Autodesk Fusion 360 part; units mm, degrees
(part 2 of 3)
  line L695 (-16.549, 126.6806) -> (-16.4532, 126.8438)
  line L696 (-16.4532, 126.8438) -> (-16.3127, 126.9927)
  line L697 (-16.3127, 126.9927) -> (-16.1723, 127.1416)
  line L698 (-16.1723, 127.1416) -> (-16.0457, 127.2313)
  spline S85 degree 3 poles (-16.0457, 127.2313) (-15.8814, 127.3478) (-15.7503, 127.4125) (-15.5307, 127.4855) knots 0 0 0 0 1 1 1 1
  line L699 (-15.5307, 127.4855) -> (-15.3521, 127.5448)
  line L700 (-15.3521, 127.5448) -> (-14.9951, 127.5456)
  line L701 (-14.9951, 127.5456) -> (-14.6381, 127.5465)
  line L702 (-14.6381, 127.5465) -> (-14.4281, 127.4721)
  line L703 (-14.4281, 127.4721) -> (-14.2181, 127.3978)
  line L704 (-14.2181, 127.3978) -> (-8.7577, 124.2519)
  spline S86 degree 3 poles (-8.7577, 124.2519) (-5.7545, 122.5216) (-3.2454, 121.0723) (-3.1819, 121.0312) knots 0 0 0 0 1 1 1 1
  line L705 (-3.1819, 121.0312) -> (-3.0664, 120.9565)
  line L706 (-3.0664, 120.9565) -> (-2.9089, 120.7961)
  line L707 (-2.9089, 120.7961) -> (-2.7514, 120.6356)
  line L708 (-2.7514, 120.6356) -> (-2.6525, 120.4684)
  line L709 (-2.6525, 120.4684) -> (-2.5536, 120.3011)
  line L710 (-2.5536, 120.3011) -> (-2.4864, 120.1016)
  line L711 (-2.4864, 120.1016) -> (-2.4191, 119.9021)
  line L712 (-2.4191, 119.9021) -> (-2.4097, 119.608)
  line L713 (-2.4097, 119.608) -> (-2.4003, 119.314)
  line L714 (-2.4003, 119.314) -> (-2.4444, 119.1292)
  line L715 (-2.4444, 119.1292) -> (-2.4886, 118.9443)
  line L716 (-2.4886, 118.9443) -> (-2.5601, 118.7895)
  spline S87 degree 3 poles (-2.5601, 118.7895) (-2.6533, 118.5878) (-2.7387, 118.4645) (-2.9076, 118.2878) knots 0 0 0 0 1 1 1 1
  line L717 (-2.9076, 118.2878) -> (-3.0454, 118.1436)
  line L718 (-3.0454, 118.1436) -> (-3.1674, 118.0604)
  spline S88 degree 3 poles (-3.1674, 118.0604) (-3.3211, 117.9556) (-3.554, 117.8452) (-3.7174, 117.7997) knots 0 0 0 0 1 1 1 1
  line L719 (-3.7174, 117.7997) -> (-3.8434, 117.7647)
  line L720 (-3.8434, 117.7647) -> (-4.1584, 117.7571)
  line L721 (-4.1584, 117.7571) -> (-4.4735, 117.7496)
  line L722 (-4.4735, 117.7496) -> (-4.625, 117.7904)
  spline S89 degree 3 poles (-3.8806, 117.8246) (-3.6716, 117.8678) (-3.4777, 117.9415) (-3.3069, 118.0427) knots 0 0 0 0 1 1 1 1
  line L723 (-3.3069, 118.0427) -> (-3.1695, 118.1242)
  line L724 (-3.1695, 118.1242) -> (-3.0182, 118.2642)
  line L725 (-3.0182, 118.2642) -> (-2.867, 118.4043)
  line L726 (-2.867, 118.4043) -> (-2.7535, 118.5756)
  line L727 (-2.7535, 118.5756) -> (-2.64, 118.747)
  line L728 (-2.64, 118.747) -> (-2.5873, 118.8731)
  spline S90 degree 3 poles (-2.5873, 118.8731) (-2.5584, 118.9424) (-2.5191, 119.0592) (-2.5001, 119.1327) knots 0 0 0 0 1 1 1 1
  line L729 (-2.5001, 119.1327) -> (-2.4655, 119.2663)
  line L730 (-2.4655, 119.2663) -> (-2.4531, 119.4414)
  line L731 (-2.4531, 119.4414) -> (-2.4407, 119.6165)
  line L732 (-2.4407, 119.6165) -> (-2.4666, 119.7766)
  line L733 (-2.4666, 119.7766) -> (-2.4924, 119.9366)
  line L734 (-2.4924, 119.9366) -> (-2.543, 120.0853)
  spline S91 degree 3 poles (-2.543, 120.0853) (-2.666, 120.4472) (-2.9021, 120.7612) (-3.2134, 120.9768) knots 0 0 0 0 1 1 1 1
  spline S92 degree 3 poles (-3.2134, 120.9768) (-3.2973, 121.035) (-14.1137, 127.2678) (-14.2431, 127.3327) knots 0 0 0 0 1 1 1 1
  spline S93 degree 3 poles (-14.2431, 127.3327) (-14.3718, 127.3971) (-14.5821, 127.4647) (-14.7417, 127.493) knots 0 0 0 0 1 1 1 1
  line L735 (-14.7417, 127.493) -> (-14.8663, 127.515)
  line L736 (-14.8663, 127.515) -> (-15.0042, 127.5148)
  line L737 (-15.0042, 127.5148) -> (-15.1421, 127.5145)
  line L738 (-15.1421, 127.5145) -> (-15.3388, 127.4739)
  line L739 (-15.3388, 127.4739) -> (-15.5355, 127.4333)
  line L740 (-15.5355, 127.4333) -> (-15.7483, 127.3288)
  line L741 (-15.7483, 127.3288) -> (-15.9612, 127.2242)
  line L742 (-15.9612, 127.2242) -> (-16.0864, 127.1225)
  line L743 (-16.0864, 127.1225) -> (-16.2117, 127.0208)
  line L744 (-16.2117, 127.0208) -> (-16.3352, 126.8742)
  line L745 (-16.3352, 126.8742) -> (-16.4587, 126.7275)
  line L746 (-16.4587, 126.7275) -> (-16.5605, 126.5175)
  line L747 (-16.5605, 126.5175) -> (-16.6624, 126.3075)
  line L748 (-16.6624, 126.3075) -> (-16.699, 126.171)
  line L749 (-16.699, 126.171) -> (-16.7357, 126.0344)
  line L750 (-16.7357, 126.0344) -> (-16.7365, 125.7719)
  line L751 (-16.7365, 125.7719) -> (-16.7373, 125.5094)
  line L752 (-16.7373, 125.5094) -> (-16.6987, 125.3624)
  line L753 (-16.6987, 125.3624) -> (-16.6601, 125.2154)
  line L754 (-16.6601, 125.2154) -> (-16.5778, 125.038)
  line L755 (-16.5778, 125.038) -> (-16.4955, 124.8605)
  line L756 (-16.4955, 124.8605) -> (-16.3808, 124.7081)
  line L757 (-16.3808, 124.7081) -> (-16.2661, 124.5557)
  line L758 (-16.2661, 124.5557) -> (-16.1449, 124.455)
  spline S94 degree 3 poles (-16.1449, 124.455) (-16.0783, 124.3997) (-15.9766, 124.3246) (-15.9189, 124.2882) knots 0 0 0 0 1 1 1 1
  spline S95 degree 3 poles (-15.9189, 124.2882) (-15.8613, 124.2519) (-13.3806, 122.8204) (-10.4063, 121.1072) knots 0 0 0 0 1 1 1 1
  line L759 (-10.4063, 121.1072) -> (-4.9985, 117.9923)
  line L760 (-4.9985, 117.9923) -> (-4.841, 117.9247)
  line L761 (-4.841, 117.9247) -> (-4.6835, 117.857)
  line L762 (-4.6835, 117.857) -> (-4.5365, 117.8259)
  line L763 (-4.5365, 117.8259) -> (-4.3895, 117.7949)
  line L764 (-4.3895, 117.7949) -> (-4.2153, 117.7931)
  line L765 (-4.2153, 117.7931) -> (-4.0412, 117.7914)
  line L766 (-4.0412, 117.7914) -> (-3.8806, 117.8246)
  spline S96 degree 3 poles (3.4229, 117.7903) (3.342, 117.8116) (3.2176, 117.8526) (3.1465, 117.8815) knots 0 0 0 0 1 1 1 1
  line L767 (3.1465, 117.8815) -> (3.0173, 117.934)
  line L768 (3.0173, 117.934) -> (2.8685, 118.0302)
  line L769 (2.8685, 118.0302) -> (2.7197, 118.1265)
  line L770 (2.7197, 118.1265) -> (2.5826, 118.2636)
  line L771 (2.5826, 118.2636) -> (2.4455, 118.4007)
  line L772 (2.4455, 118.4007) -> (2.3421, 118.559)
  line L773 (2.3421, 118.559) -> (2.2388, 118.7173)
  line L774 (2.2388, 118.7173) -> (2.1937, 118.8371)
  spline S97 degree 3 poles (2.1937, 118.8371) (2.1689, 118.9031) (2.1298, 119.0279) (2.1069, 119.1145) knots 0 0 0 0 1 1 1 1
  line L775 (2.1069, 119.1145) -> (2.0652, 119.272)
  line L776 (2.0652, 119.272) -> (2.0654, 119.545)
  line L777 (2.0654, 119.545) -> (2.0657, 119.8181)
  line L778 (2.0657, 119.8181) -> (2.1094, 119.9861)
  line L779 (2.1094, 119.9861) -> (2.1531, 120.1541)
  line L780 (2.1531, 120.1541) -> (2.2252, 120.3062)
  spline S98 degree 3 poles (2.2252, 120.3062) (2.3166, 120.4993) (2.4034, 120.6261) (2.5503, 120.7813) knots 0 0 0 0 1 1 1 1
  line L781 (2.5503, 120.7813) -> (2.667, 120.9046)
  line L782 (2.667, 120.9046) -> (2.793, 120.9942)
  spline S99 degree 3 poles (2.793, 120.9942) (2.9532, 121.1083) (13.7543, 127.3341) (13.9237, 127.41) knots 0 0 0 0 1 1 1 1
  spline S100 degree 3 poles (13.9237, 127.41) (13.993, 127.4411) (14.1111, 127.4845) (14.1862, 127.5065) knots 0 0 0 0 1 1 1 1
  line L783 (14.1862, 127.5065) -> (14.3227, 127.5465)
  line L784 (14.3227, 127.5465) -> (14.6692, 127.5459)
  line L785 (14.6692, 127.5459) -> (15.0157, 127.5453)
  line L786 (15.0157, 127.5453) -> (15.2204, 127.4751)
  line L787 (15.2204, 127.4751) -> (15.425, 127.4048)
  line L788 (15.425, 127.4048) -> (15.5943, 127.3006)
  line L789 (15.5943, 127.3006) -> (15.7635, 127.1965)
  line L790 (15.7635, 127.1965) -> (15.9006, 127.0683)
  line L791 (15.9006, 127.0683) -> (16.0377, 126.94)
  line L792 (16.0377, 126.94) -> (16.1605, 126.7535)
  line L793 (16.1605, 126.7535) -> (16.2834, 126.567)
  line L794 (16.2834, 126.567) -> (16.3455, 126.3952)
  line L795 (16.3455, 126.3952) -> (16.4076, 126.2235)
  line L796 (16.4076, 126.2235) -> (16.4339, 126.0605)
  line L797 (16.4339, 126.0605) -> (16.4602, 125.8975)
  line L798 (16.4602, 125.8975) -> (16.448, 125.6614)
  line L799 (16.448, 125.6614) -> (16.4358, 125.4254)
  line L800 (16.4358, 125.4254) -> (16.4014, 125.2994)
  line L801 (16.4014, 125.2994) -> (16.3671, 125.1734)
  line L802 (16.3671, 125.1734) -> (16.2777, 124.9844)
  line L803 (16.2777, 124.9844) -> (16.1883, 124.7954)
  line L804 (16.1883, 124.7954) -> (16.062, 124.637)
  line L805 (16.062, 124.637) -> (15.9357, 124.4786)
  line L806 (15.9357, 124.4786) -> (15.8012, 124.3717)
  line L807 (15.8012, 124.3717) -> (15.6668, 124.2649)
  line L808 (15.6668, 124.2649) -> (10.2064, 121.1194)
  spline S101 degree 3 poles (10.2064, 121.1194) (7.2032, 119.3894) (4.6799, 117.9425) (4.5991, 117.904) knots 0 0 0 0 1 1 1 1
  line L809 (4.5991, 117.904) -> (4.4521, 117.8341)
  line L810 (4.4521, 117.8341) -> (4.286, 117.7918)
  line L811 (4.286, 117.7918) -> (4.1198, 117.7494)
  line L812 (4.1198, 117.7494) -> (3.8449, 117.7506)
  line L813 (3.8449, 117.7506) -> (3.57, 117.7518)
  line L814 (3.57, 117.7518) -> (3.4229, 117.7903)
  spline S102 degree 3 poles (4.151, 117.8211) (4.2357, 117.8375) (4.3676, 117.8737) (4.4441, 117.9015) knots 0 0 0 0 1 1 1 1
  line L815 (4.4441, 117.9015) -> (4.5831, 117.9522)
  line L816 (4.5831, 117.9522) -> (10.083, 121.1192)
  line L817 (10.083, 121.1192) -> (15.5828, 124.2861)
  line L818 (15.5828, 124.2861) -> (15.6884, 124.3646)
  spline S103 degree 3 poles (15.6884, 124.3646) (15.7465, 124.4078) (15.8441, 124.4941) (15.9054, 124.5563) knots 0 0 0 0 1 1 1 1
  line L819 (15.9054, 124.5563) -> (16.0168, 124.6694)
  line L820 (16.0168, 124.6694) -> (16.1204, 124.8264)
  line L821 (16.1204, 124.8264) -> (16.2239, 124.9833)
  line L822 (16.2239, 124.9833) -> (16.2864, 125.1454)
  line L823 (16.2864, 125.1454) -> (16.3489, 125.3075)
  line L824 (16.3489, 125.3075) -> (16.3829, 125.5029)
  line L825 (16.3829, 125.5029) -> (16.4168, 125.6984)
  line L826 (16.4168, 125.6984) -> (16.4028, 125.8737)
  line L827 (16.4028, 125.8737) -> (16.3888, 126.0489)
  line L828 (16.3888, 126.0489) -> (16.3363, 126.2307)
  line L829 (16.3363, 126.2307) -> (16.2839, 126.4125)
  line L830 (16.2839, 126.4125) -> (16.1992, 126.57)
  line L831 (16.1992, 126.57) -> (16.1145, 126.7275)
  line L832 (16.1145, 126.7275) -> (16.0024, 126.8662)
  line L833 (16.0024, 126.8662) -> (15.8904, 127.0049)
  line L834 (15.8904, 127.0049) -> (15.756, 127.1119)
  line L835 (15.756, 127.1119) -> (15.6216, 127.2188)
  line L836 (15.6216, 127.2188) -> (15.4657, 127.3016)
  spline S104 degree 3 poles (15.4657, 127.3016) (15.2046, 127.4402) (14.9145, 127.5149) (14.6377, 127.5146) knots 0 0 0 0 1 1 1 1
  line L837 (14.6377, 127.5146) -> (14.5117, 127.5145)
  line L838 (14.5117, 127.5145) -> (14.3139, 127.4737)
  line L839 (14.3139, 127.4737) -> (14.1161, 127.4328)
  line L840 (14.1161, 127.4328) -> (13.9464, 127.3511)
  spline S105 degree 3 poles (13.9464, 127.3511) (13.853, 127.3062) (11.3296, 125.8591) (8.3388, 124.1353) knots 0 0 0 0 1 1 1 1
  line L841 (8.3388, 124.1353) -> (2.9009, 121.0012)
  line L842 (2.9009, 121.0012) -> (2.7814, 120.9093)
  spline S106 degree 3 poles (2.7814, 120.9093) (2.6252, 120.7891) (2.4901, 120.6371) (2.3742, 120.4511) knots 0 0 0 0 1 1 1 1
  line L843 (2.3742, 120.4511) -> (2.2803, 120.3006)
  line L844 (2.2803, 120.3006) -> (2.2286, 120.163)
  spline S107 degree 3 poles (2.2286, 120.163) (2.2001, 120.0873) (2.1619, 119.9532) (2.1436, 119.8649) knots 0 0 0 0 1 1 1 1
  line L845 (2.1436, 119.8649) -> (2.1105, 119.7043)
  line L846 (2.1105, 119.7043) -> (2.1105, 119.5345)
  line L847 (2.1105, 119.5345) -> (2.1105, 119.3648)
  line L848 (2.1105, 119.3648) -> (2.1437, 119.2029)
  line L849 (2.1437, 119.2029) -> (2.177, 119.041)
  line L850 (2.177, 119.041) -> (2.2399, 118.8894)
  spline S108 degree 3 poles (2.2399, 118.8894) (2.2745, 118.806) (2.3408, 118.6784) (2.3871, 118.6059) knots 0 0 0 0 1 1 1 1
  line L851 (2.3871, 118.6059) -> (2.4713, 118.474)
  line L852 (2.4713, 118.474) -> (2.6112, 118.3304)
  line L853 (2.6112, 118.3304) -> (2.751, 118.1867)
  line L854 (2.751, 118.1867) -> (2.8665, 118.1075)
  spline S109 degree 3 poles (2.8665, 118.1075) (3.1626, 117.9043) (3.4886, 117.7988) (3.836, 117.7938) knots 0 0 0 0 1 1 1 1
  line L855 (3.836, 117.7938) -> (3.9969, 117.7914)
  line L856 (3.9969, 117.7914) -> (4.151, 117.8211)
  spline S110 degree 3 poles (-0.3677, 120.0717) (-0.3966, 120.0769) (-0.4769, 120.0913) (-0.5462, 120.1038) knots 0 0 0 0 1 1 1 1
  line L857 (-0.5462, 120.1038) -> (-0.6722, 120.1264)
  line L858 (-0.6722, 120.1264) -> (-0.8328, 120.1882)
  line L859 (-0.8328, 120.1882) -> (-0.9933, 120.2499)
  line L860 (-0.9933, 120.2499) -> (-1.1268, 120.3362)
  spline S111 degree 3 poles (-1.1268, 120.3362) (-1.2002, 120.3836) (-1.3095, 120.4645) (-1.3697, 120.5159) knots 0 0 0 0 1 1 1 1
  line L861 (-1.3697, 120.5159) -> (-1.4792, 120.6094)
  line L862 (-1.4792, 120.6094) -> (-1.594, 120.7598)
  line L863 (-1.594, 120.7598) -> (-1.7088, 120.9101)
  line L864 (-1.7088, 120.9101) -> (-1.7932, 121.0853)
  line L865 (-1.7932, 121.0853) -> (-1.8777, 121.2605)
  line L866 (-1.8777, 121.2605) -> (-1.9215, 121.4529)
  line L867 (-1.9215, 121.4529) -> (-1.9653, 121.6452)
  line L868 (-1.9653, 121.6452) -> (-1.9593, 128.1661)
  line L869 (-1.9593, 128.1661) -> (-1.9533, 134.687)
  line L870 (-1.9533, 134.687) -> (-1.8855, 134.8865)
  line L871 (-1.8855, 134.8865) -> (-1.8178, 135.086)
  line L872 (-1.8178, 135.086) -> (-1.7215, 135.25)
  line L873 (-1.7215, 135.25) -> (-1.6253, 135.414)
  line L874 (-1.6253, 135.414) -> (-1.4762, 135.571)
  line L875 (-1.4762, 135.571) -> (-1.327, 135.728)
  line L876 (-1.327, 135.728) -> (-1.176, 135.829)
  line L877 (-1.176, 135.829) -> (-1.0249, 135.9301)
  line L878 (-1.0249, 135.9301) -> (-0.8696, 135.9947)
  line L879 (-0.8696, 135.9947) -> (-0.7142, 136.0593)
  line L880 (-0.7142, 136.0593) -> (-0.5374, 136.095)
  line L881 (-0.5374, 136.095) -> (-0.3606, 136.1308)
  line L882 (-0.3606, 136.1308) -> (-0.0859, 136.1208)
  line L883 (-0.0859, 136.1208) -> (0.1888, 136.1107)
  line L884 (0.1888, 136.1107) -> (0.3935, 136.042)
  line L885 (0.3935, 136.042) -> (0.5981, 135.9733)
  line L886 (0.5981, 135.9733) -> (0.7647, 135.8708)
  line L887 (0.7647, 135.8708) -> (0.9313, 135.7683)
  line L888 (0.9313, 135.7683) -> (1.0477, 135.6619)
  spline S112 degree 3 poles (1.0477, 135.6619) (1.1117, 135.6034) (1.208, 135.4971) (1.2617, 135.4257) knots 0 0 0 0 1 1 1 1
  line L889 (1.2617, 135.4257) -> (1.3592, 135.296)
  line L890 (1.3592, 135.296) -> (1.4404, 135.1346)
  spline S113 degree 3 poles (1.4404, 135.1346) (1.485, 135.0459) (1.543, 134.9041) (1.5692, 134.8196) knots 0 0 0 0 1 1 1 1
  line L891 (1.5692, 134.8196) -> (1.6169, 134.666)
  line L892 (1.6169, 134.666) -> (1.6229, 128.1871)
  line L893 (1.6229, 128.1871) -> (1.6288, 121.7082)
  line L894 (1.6288, 121.7082) -> (1.6063, 121.5717)
  spline S114 degree 3 poles (1.6063, 121.5717) (1.5939, 121.4966) (1.5604, 121.3639) (1.5318, 121.2767) knots 0 0 0 0 1 1 1 1
  line L895 (1.5318, 121.2767) -> (1.4798, 121.1183)
  line L896 (1.4798, 121.1183) -> (1.3844, 120.9552)
  line L897 (1.3844, 120.9552) -> (1.2889, 120.7921)
  line L898 (1.2889, 120.7921) -> (1.1399, 120.6353)
  spline S115 degree 3 poles (1.1399, 120.6353) (0.9592, 120.445) (0.8438, 120.3584) (0.6271, 120.2501) knots 0 0 0 0 1 1 1 1
  line L899 (0.6271, 120.2501) -> (0.4619, 120.1676)
  line L900 (0.4619, 120.1676) -> (0.2938, 120.1235)
  line L901 (0.2938, 120.1235) -> (0.1258, 120.0794)
  line L902 (0.1258, 120.0794) -> (-0.0947, 120.0709)
  spline S116 degree 3 poles (-0.0947, 120.0709) (-0.216, 120.0662) (-0.3388, 120.0666) (-0.3677, 120.0717) knots 0 0 0 0 1 1 1 1
  line L903 (0.2165, 120.1648) -> (0.3912, 120.2066)
  line L904 (0.3912, 120.2066) -> (0.5457, 120.278)
  spline S117 degree 3 poles (0.5457, 120.278) (0.7389, 120.3673) (0.8685, 120.4553) (1.0261, 120.6045) knots 0 0 0 0 1 1 1 1
  line L905 (1.0261, 120.6045) -> (1.1493, 120.7211)
  line L906 (1.1493, 120.7211) -> (1.2389, 120.8471)
  spline S118 degree 3 poles (1.2389, 120.8471) (1.3602, 121.0178) (1.4477, 121.1975) (1.517, 121.4184) knots 0 0 0 0 1 1 1 1
  line L907 (1.517, 121.4184) -> (1.5749, 121.6032)
  line L908 (1.5749, 121.6032) -> (1.5749, 128.0821)
  line L909 (1.5749, 128.0821) -> (1.5749, 134.561)
  line L910 (1.5749, 134.561) -> (1.5278, 134.7376)
  line L911 (1.5278, 134.7376) -> (1.4807, 134.9143)
  line L912 (1.4807, 134.9143) -> (1.3974, 135.0842)
  line L913 (1.3974, 135.0842) -> (1.3141, 135.254)
  line L914 (1.3141, 135.254) -> (1.2048, 135.3982)
  line L915 (1.2048, 135.3982) -> (1.0954, 135.5423)
  line L916 (1.0954, 135.5423) -> (0.9572, 135.6569)
  spline S119 degree 3 poles (0.9572, 135.6569) (0.7085, 135.863) (0.4228, 135.9976) (0.1153, 136.0535) knots 0 0 0 0 1 1 1 1
  line L917 (0.1153, 136.0535) -> (-0.0422, 136.0821)
  line L918 (-0.0422, 136.0821) -> (-0.1787, 136.0826)
  line L919 (-0.1787, 136.0826) -> (-0.3152, 136.0831)
  line L920 (-0.3152, 136.0831) -> (-0.5147, 136.0422)
  line L921 (-0.5147, 136.0422) -> (-0.7142, 136.0013)
  line L922 (-0.7142, 136.0013) -> (-0.9242, 135.8966)
  line L923 (-0.9242, 135.8966) -> (-1.1342, 135.7918)
  line L924 (-1.1342, 135.7918) -> (-1.2665, 135.684)
  line L925 (-1.2665, 135.684) -> (-1.3987, 135.5761)
  line L926 (-1.3987, 135.5761) -> (-1.5149, 135.4361)
  line L927 (-1.5149, 135.4361) -> (-1.6311, 135.2961)
  line L928 (-1.6311, 135.2961) -> (-1.7356, 135.0832)
  line L929 (-1.7356, 135.0832) -> (-1.8401, 134.8704)
  line L930 (-1.8401, 134.8704) -> (-1.8807, 134.6737)
  line L931 (-1.8807, 134.6737) -> (-1.9212, 134.477)
  line L932 (-1.9212, 134.477) -> (-1.9214, 128.1136)
  line L933 (-1.9214, 128.1136) -> (-1.9216, 121.7502)
  line L934 (-1.9216, 121.7502) -> (-1.8994, 121.6137)
  spline S120 degree 3 poles (-1.8994, 121.6137) (-1.8873, 121.5386) (-1.8538, 121.4063) (-1.8249, 121.3197) knots 0 0 0 0 1 1 1 1
  line L935 (-1.8249, 121.3197) -> (-1.7725, 121.1622)
  line L936 (-1.7725, 121.1622) -> (-1.6845, 121.0047)
  line L937 (-1.6845, 121.0047) -> (-1.5964, 120.8472)
  line L938 (-1.5964, 120.8472) -> (-1.3968, 120.6454)
  line L939 (-1.3968, 120.6454) -> (-1.1973, 120.4437)
  line L940 (-1.1973, 120.4437) -> (-1.0515, 120.3631)
  spline S121 degree 3 poles (-1.0515, 120.3631) (-0.8617, 120.2581) (-0.688, 120.1888) (-0.5281, 120.154) knots 0 0 0 0 1 1 1 1
  line L941 (-0.5281, 120.154) -> (-0.3993, 120.126)
  line L942 (-0.3993, 120.126) -> (-0.1788, 120.1244)
  line L943 (-0.1788, 120.1244) -> (0.0417, 120.1229)
  line L944 (0.0417, 120.1229) -> (0.2165, 120.1648)
  line L945 (-15.2447, 128.6299) -> (-15.3892, 128.6495)
  line L946 (-15.3892, 128.6495) -> (-15.5775, 128.7126)
  line L947 (-15.5775, 128.7126) -> (-15.7659, 128.7757)
  line L948 (-15.7659, 128.7757) -> (-15.9055, 128.8578)
  spline S122 degree 3 poles (-15.9055, 128.8578) (-16.226, 129.046) (-16.4764, 129.324) (-16.6354, 129.6682) knots 0 0 0 0 1 1 1 1
  line L949 (-16.6354, 129.6682) -> (-16.707, 129.823)
  line L950 (-16.707, 129.823) -> (-16.751, 130.0079)
  line L951 (-16.751, 130.0079) -> (-16.795, 130.1927)
  line L952 (-16.795, 130.1927) -> (-16.785, 130.4762)
  line L953 (-16.785, 130.4762) -> (-16.775, 130.7597)
  line L954 (-16.775, 130.7597) -> (-16.7403, 130.8857)
  spline S123 degree 3 poles (-16.7403, 130.8857) (-16.7212, 130.9551) (-16.6675, 131.0921) (-16.6208, 131.1903) knots 0 0 0 0 1 1 1 1
  line L955 (-16.6208, 131.1903) -> (-16.536, 131.3688)
  line L956 (-16.536, 131.3688) -> (-16.4211, 131.5192)
  line L957 (-16.4211, 131.5192) -> (-16.3061, 131.6695)
  line L958 (-16.3061, 131.6695) -> (-16.1966, 131.7629)
  spline S124 degree 3 poles (-16.1966, 131.7629) (-16.1364, 131.8143) (-16.0352, 131.8892) (-15.9717, 131.9293) knots 0 0 0 0 1 1 1 1
  spline S125 degree 3 poles (-15.9717, 131.9293) (-15.9081, 131.9695) (-13.4046, 133.4185) (-10.4082, 135.1493) knots 0 0 0 0 1 1 1 1
  line L959 (-10.4082, 135.1493) -> (-4.9603, 138.2963)
  line L960 (-4.9603, 138.2963) -> (-4.7841, 138.3555)
  line L961 (-4.7841, 138.3555) -> (-4.6079, 138.4147)
  line L962 (-4.6079, 138.4147) -> (-4.2011, 138.4147)
  line L963 (-4.2011, 138.4147) -> (-3.7943, 138.4147)
  line L964 (-3.7943, 138.4147) -> (-3.6088, 138.3494)
  line L965 (-3.6088, 138.3494) -> (-3.4234, 138.2841)
  line L966 (-3.4234, 138.2841) -> (-3.2793, 138.2001)
  line L967 (-3.2793, 138.2001) -> (-3.1351, 138.1161)
  line L968 (-3.1351, 138.1161) -> (-2.9774, 137.9662)
  line L969 (-2.9774, 137.9662) -> (-2.8196, 137.8164)
  line L970 (-2.8196, 137.8164) -> (-2.7302, 137.6903)
  spline S126 degree 3 poles (-2.7302, 137.6903) (-2.6139, 137.5261) (-2.5492, 137.3948) (-2.4767, 137.1756) knots 0 0 0 0 1 1 1 1
  line L971 (-2.4767, 137.1756) -> (-2.4176, 136.9971)
  line L972 (-2.4176, 136.9971) -> (-2.4165, 136.6716)
  line L973 (-2.4165, 136.6716) -> (-2.4153, 136.3461)
  line L974 (-2.4153, 136.3461) -> (-2.4523, 136.2121)
  spline S127 degree 3 poles (-2.4523, 136.2121) (-2.5025, 136.0305) (-2.5753, 135.8544) (-2.6599, 135.7102) knots 0 0 0 0 1 1 1 1
  line L975 (-2.6599, 135.7102) -> (-2.7303, 135.59)
  line L976 (-2.7303, 135.59) -> (-2.9404, 135.38)
  line L977 (-2.9404, 135.38) -> (-3.1504, 135.17)
  line L978 (-3.1504, 135.17) -> (-8.6354, 132.0037)
  spline S128 degree 3 poles (-8.6354, 132.0037) (-11.6521, 130.2623) (-14.1801, 128.8094) (-14.2532, 128.7752) knots 0 0 0 0 1 1 1 1
  line L979 (-14.2532, 128.7752) -> (-14.3861, 128.7131)
  line L980 (-14.3861, 128.7131) -> (-14.5436, 128.6729)
  line L981 (-14.5436, 128.6729) -> (-14.7011, 128.6327)
  line L982 (-14.7011, 128.6327) -> (-14.9006, 128.6215)
  line L983 (-14.9006, 128.6215) -> (-15.1001, 128.6103)
  line L984 (-15.1001, 128.6103) -> (-15.2447, 128.6299)
  line L985 (-14.4687, 128.7571) -> (-14.2573, 128.8298)
  line L986 (-14.2573, 128.8298) -> (-8.8089, 131.9757)
  spline S129 degree 3 poles (-8.8089, 131.9757) (-5.8122, 133.7059) (-3.3084, 135.1553) (-3.2449, 135.1966) knots 0 0 0 0 1 1 1 1
  spline S130 degree 3 poles (-3.2449, 135.1966) (-3.1814, 135.238) (-3.0739, 135.3245) (-3.0062, 135.3889) knots 0 0 0 0 1 1 1 1
  line L987 (-3.0062, 135.3889) -> (-2.8829, 135.506)
  line L988 (-2.8829, 135.506) -> (-2.7904, 135.6353)
  line L989 (-2.7904, 135.6353) -> (-2.698, 135.7646)
  line L990 (-2.698, 135.7646) -> (-2.6167, 135.9398)
  line L991 (-2.6167, 135.9398) -> (-2.5355, 136.1151)
  line L992 (-2.5355, 136.1151) -> (-2.4975, 136.2621)
  line L993 (-2.4975, 136.2621) -> (-2.4596, 136.4091)
  line L994 (-2.4596, 136.4091) -> (-2.4596, 136.6506)
  line L995 (-2.4596, 136.6506) -> (-2.4596, 136.8921)
  line L996 (-2.4596, 136.8921) -> (-2.4975, 137.0391)
  line L997 (-2.4975, 137.0391) -> (-2.5355, 137.1861)
  line L998 (-2.5355, 137.1861) -> (-2.6167, 137.3614)
  line L999 (-2.6167, 137.3614) -> (-2.698, 137.5366)
  line L1000 (-2.698, 137.5366) -> (-2.7904, 137.6659)
  line L1001 (-2.7904, 137.6659) -> (-2.8829, 137.7952)
  line L1002 (-2.8829, 137.7952) -> (-3.0062, 137.9118)
  spline S131 degree 3 poles (-3.0062, 137.9118) (-3.1638, 138.0609) (-3.2933, 138.149) (-3.4866, 138.2383) knots 0 0 0 0 1 1 1 1
  line L1003 (-3.4866, 138.2383) -> (-3.6411, 138.3097)
  line L1004 (-3.6411, 138.3097) -> (-3.8157, 138.3515)
  line L1005 (-3.8157, 138.3515) -> (-3.9904, 138.3934)
  line L1006 (-3.9904, 138.3934) -> (-4.2004, 138.3934)
  line L1007 (-4.2004, 138.3934) -> (-4.4105, 138.3934)
  line L1008 (-4.4105, 138.3934) -> (-4.5832, 138.352)
  line L1009 (-4.5832, 138.352) -> (-4.756, 138.3106)
  line L1010 (-4.756, 138.3106) -> (-4.8877, 138.2508)
  spline S132 degree 3 poles (-4.8877, 138.2508) (-5.059, 138.173) (-15.8375, 131.9473) (-16.0037, 131.8301) knots 0 0 0 0 1 1 1 1
  line L1011 (-16.0037, 131.8301) -> (-16.1302, 131.7409)
  line L1012 (-16.1302, 131.7409) -> (-16.2696, 131.5932)
  line L1013 (-16.2696, 131.5932) -> (-16.4089, 131.4455)
  line L1014 (-16.4089, 131.4455) -> (-16.4975, 131.2965)
  line L1015 (-16.4975, 131.2965) -> (-16.586, 131.1474)
  line L1016 (-16.586, 131.1474) -> (-16.6455, 130.9746)
  line L1017 (-16.6455, 130.9746) -> (-16.7049, 130.8017)
  line L1018 (-16.7049, 130.8017) -> (-16.7294, 130.6442)
  line L1019 (-16.7294, 130.6442) -> (-16.7539, 130.4867)
  line L1020 (-16.7539, 130.4867) -> (-16.742, 130.3158)
  line L1021 (-16.742, 130.3158) -> (-16.7301, 130.1449)
  line L1022 (-16.7301, 130.1449) -> (-16.6955, 130.0114)
  spline S133 degree 3 poles (-16.6955, 130.0114) (-16.6465, 129.8223) (-16.5698, 129.6488) (-16.4605, 129.4797) knots 0 0 0 0 1 1 1 1
  line L1023 (-16.4605, 129.4797) -> (-16.3661, 129.3337)
  line L1024 (-16.3661, 129.3337) -> (-16.2372, 129.1994)
  line L1025 (-16.2372, 129.1994) -> (-16.1082, 129.0652)
  line L1026 (-16.1082, 129.0652) -> (-15.959, 128.9654)
  line L1027 (-15.959, 128.9654) -> (-15.8099, 128.8656)
  line L1028 (-15.8099, 128.8656) -> (-15.6545, 128.801)
  line L1029 (-15.6545, 128.801) -> (-15.4991, 128.7364)
  line L1030 (-15.4991, 128.7364) -> (-15.3521, 128.7036)
  line L1031 (-15.3521, 128.7036) -> (-15.2051, 128.6709)
  line L1032 (-15.2051, 128.6709) -> (-14.9426, 128.6777)
  line L1033 (-14.9426, 128.6777) -> (-14.6801, 128.6844)
  line L1034 (-14.6801, 128.6844) -> (-14.4687, 128.7571)
  line L1035 (14.4092, 128.6299) -> (14.2646, 128.6495)
  line L1036 (14.2646, 128.6495) -> (14.0759, 128.7128)
  line L1037 (14.0759, 128.7128) -> (13.8871, 128.776)
  line L1038 (13.8871, 128.776) -> (12.8553, 129.3717)
  spline S134 degree 3 poles (12.8553, 129.3717) (12.2879, 129.6993) (9.8025, 131.1353) (7.3323, 132.5627) knots 0 0 0 0 1 1 1 1
  line L1039 (7.3323, 132.5627) -> (2.841, 135.1581)
  line L1040 (2.841, 135.1581) -> (2.7225, 135.2547)
  spline S135 degree 3 poles (2.7225, 135.2547) (2.6573, 135.3078) (2.5497, 135.4145) (2.4833, 135.4917) knots 0 0 0 0 1 1 1 1
  line L1041 (2.4833, 135.4917) -> (2.3627, 135.632)
  line L1042 (2.3627, 135.632) -> (2.2573, 135.8421)
  line L1043 (2.2573, 135.8421) -> (2.152, 136.0521)
  line L1044 (2.152, 136.0521) -> (2.1155, 136.1886)
  line L1045 (2.1155, 136.1886) -> (2.079, 136.3251)
  line L1046 (2.079, 136.3251) -> (2.079, 136.6611)
  line L1047 (2.079, 136.6611) -> (2.079, 136.9971)
  line L1048 (2.079, 136.9971) -> (2.1282, 137.1546)
  line L1049 (2.1282, 137.1546) -> (2.1774, 137.3121)
  line L1050 (2.1774, 137.3121) -> (2.27, 137.4907)
  line L1051 (2.27, 137.4907) -> (2.3625, 137.6692)
  line L1052 (2.3625, 137.6692) -> (2.4862, 137.818)
  line L1053 (2.4862, 137.818) -> (2.6098, 137.9669)
  line L1054 (2.6098, 137.9669) -> (2.7539, 138.075)
  spline S136 degree 3 poles (2.7539, 138.075) (2.9374, 138.2127) (3.0874, 138.2926) (3.2902, 138.3606) knots 0 0 0 0 1 1 1 1
  line L1055 (3.2902, 138.3606) -> (3.4514, 138.4147)
  line L1056 (3.4514, 138.4147) -> (3.8498, 138.4147)
  line L1057 (3.8498, 138.4147) -> (4.2482, 138.4147)
  line L1058 (4.2482, 138.4147) -> (4.3921, 138.3709)
  line L1059 (4.3921, 138.3709) -> (4.5361, 138.3271)
  line L1060 (4.5361, 138.3271) -> (4.7041, 138.2381)
  spline S137 degree 3 poles (4.7041, 138.2381) (4.967, 138.099) (15.5687, 131.9707) (15.6983, 131.883) knots 0 0 0 0 1 1 1 1
  line L1061 (15.6983, 131.883) -> (15.8138, 131.8048)
  line L1062 (15.8138, 131.8048) -> (15.9648, 131.6458)
  line L1063 (15.9648, 131.6458) -> (16.1158, 131.4868)
  line L1064 (16.1158, 131.4868) -> (16.2113, 131.3237)
  line L1065 (16.2113, 131.3237) -> (16.3068, 131.1606)
  line L1066 (16.3068, 131.1606) -> (16.3587, 131.0022)
  spline S138 degree 3 poles (16.3587, 131.0022) (16.3873, 130.915) (16.4218, 130.7784) (16.4353, 130.6986) knots 0 0 0 0 1 1 1 1
  line L1067 (16.4353, 130.6986) -> (16.4598, 130.5535)
  line L1068 (16.4598, 130.5535) -> (16.4489, 130.3101)
  line L1069 (16.4489, 130.3101) -> (16.438, 130.0667)
  line L1070 (16.438, 130.0667) -> (16.3807, 129.8882)
  spline S139 degree 3 poles (16.3807, 129.8882) (16.3111, 129.6711) (16.2466, 129.5394) (16.1287, 129.3737) knots 0 0 0 0 1 1 1 1
  line L1071 (16.1287, 129.3737) -> (16.0391, 129.2476)
  line L1072 (16.0391, 129.2476) -> (15.9055, 129.1204)
  spline S140 degree 3 poles (15.9055, 129.1204) (15.7409, 128.9638) (15.6173, 128.8784) (15.4199, 128.7849) knots 0 0 0 0 1 1 1 1
  line L1073 (15.4199, 128.7849) -> (15.2678, 128.7128)
  line L1074 (15.2678, 128.7128) -> (15.1103, 128.6727)
  line L1075 (15.1103, 128.6727) -> (14.9528, 128.6327)
  line L1076 (14.9528, 128.6327) -> (14.7532, 128.6215)
  line L1077 (14.7532, 128.6215) -> (14.5537, 128.6103)
  line L1078 (14.5537, 128.6103) -> (14.4092, 128.6299)
  spline S141 degree 3 poles (14.9801, 128.7007) (15.0601, 128.7176) (15.1906, 128.7558) (15.2699, 128.7857) knots 0 0 0 0 1 1 1 1
  line L1079 (15.2699, 128.7857) -> (15.4143, 128.84)
  line L1080 (15.4143, 128.84) -> (15.568, 128.9358)
  line L1081 (15.568, 128.9358) -> (15.7218, 129.0317)
  line L1082 (15.7218, 129.0317) -> (15.8482, 129.1487)
  line L1083 (15.8482, 129.1487) -> (15.9746, 129.2657)
  line L1084 (15.9746, 129.2657) -> (16.0679, 129.3965)
  line L1085 (16.0679, 129.3965) -> (16.1612, 129.5272)
  line L1086 (16.1612, 129.5272) -> (16.2425, 129.7025)
  line L1087 (16.2425, 129.7025) -> (16.3237, 129.8777)
  line L1088 (16.3237, 129.8777) -> (16.3619, 130.0247)
  line L1089 (16.3619, 130.0247) -> (16.4001, 130.1717)
  line L1090 (16.4001, 130.1717) -> (16.3983, 130.4237)
  line L1091 (16.3983, 130.4237) -> (16.3965, 130.6757)
  line L1092 (16.3965, 130.6757) -> (16.3412, 130.8605)
  line L1093 (16.3412, 130.8605) -> (16.286, 131.0452)
  line L1094 (16.286, 131.0452) -> (16.2207, 131.1755)
  spline S142 degree 3 poles (16.2207, 131.1755) (16.1848, 131.2471) (16.1143, 131.3637) (16.0641, 131.4345) knots 0 0 0 0 1 1 1 1
  line L1095 (16.0641, 131.4345) -> (15.9729, 131.5632)
  line L1096 (15.9729, 131.5632) -> (15.8303, 131.6939)
  line L1097 (15.8303, 131.6939) -> (15.6878, 131.8247)
  line L1098 (15.6878, 131.8247) -> (15.5198, 131.9239)
  spline S143 degree 3 poles (15.5198, 131.9239) (15.4274, 131.9784) (12.9324, 133.421) (9.9754, 135.1296) knots 0 0 0 0 1 1 1 1
  line L1099 (9.9754, 135.1296) -> (4.5991, 138.2362)
  line L1100 (4.5991, 138.2362) -> (4.3891, 138.3094)
  line L1101 (4.3891, 138.3094) -> (4.1791, 138.3825)
  line L1102 (4.1791, 138.3825) -> (3.8746, 138.3828)
  line L1103 (3.8746, 138.3828) -> (3.57, 138.3832)
  line L1104 (3.57, 138.3832) -> (3.4335, 138.3467)
  line L1105 (3.4335, 138.3467) -> (3.297, 138.3101)
  line L1106 (3.297, 138.3101) -> (3.0765, 138.2007)
  line L1107 (3.0765, 138.2007) -> (2.856, 138.0912)
  line L1108 (2.856, 138.0912) -> (2.646, 137.8802)
  line L1109 (2.646, 137.8802) -> (2.436, 137.6691)
  line L1110 (2.436, 137.6691) -> (2.3655, 137.549)
  spline S144 degree 3 poles (2.3655, 137.549) (2.2813, 137.4053) (2.2082, 137.2289) (2.1624, 137.0588) knots 0 0 0 0 1 1 1 1
  line L1111 (2.1624, 137.0588) -> (2.1289, 136.9341)
  line L1112 (2.1289, 136.9341) -> (2.1169, 136.7338)
  line L1113 (2.1169, 136.7338) -> (2.1048, 136.5335)
  line L1114 (2.1048, 136.5335) -> (2.1403, 136.3584)
  spline S145 degree 3 poles (2.1403, 136.3584) (2.1858, 136.1342) (2.2581, 135.9423) (2.3658, 135.7608) knots 0 0 0 0 1 1 1 1
  line L1115 (2.3658, 135.7608) -> (2.4513, 135.6166)
  line L1116 (2.4513, 135.6166) -> (2.5974, 135.4627)
  line L1117 (2.5974, 135.4627) -> (2.7436, 135.3088)
  line L1118 (2.7436, 135.3088) -> (2.8838, 135.2147)
  spline S146 degree 3 poles (2.8838, 135.2147) (2.9609, 135.163) (5.4575, 133.7148) (8.4318, 131.9965) knots 0 0 0 0 1 1 1 1
  line L1119 (8.4318, 131.9965) -> (13.8397, 128.8724)
  line L1120 (13.8397, 128.8724) -> (13.9972, 128.804)
  line L1121 (13.9972, 128.804) -> (14.1547, 128.7357)
  line L1122 (14.1547, 128.7357) -> (14.3017, 128.7046)
  line L1123 (14.3017, 128.7046) -> (14.4487, 128.6735)
  line L1124 (14.4487, 128.6735) -> (14.6416, 128.6718)
  line L1125 (14.6416, 128.6718) -> (14.8345, 128.6701)
  line L1126 (14.8345, 128.6701) -> (14.9801, 128.7007)
  point P0 (43, 0)
  dimension "d7" = 15
  dimension "d8" = 3
  dimension "d9" = 3
  dimension "d13" = 70
  constraint horizontal L4
  constraint vertical L5
  constraint horizontal L6
  constraint vertical L7
  constraint coincident L2.end L3.start
  constraint coincident P0 L5.end
  constraint horizontal L8
  constraint vertical L9
  constraint horizontal L10
  constraint vertical L11
  constraint coincident L3 L8.start
  constraint horizontal L12
  constraint vertical L13
  constraint horizontal L14
  constraint vertical L15
  constraint coincident L7 L12.start
  constraint horizontal L16
  constraint vertical L17
  constraint horizontal L18
  constraint vertical L19
  constraint coincident L7 L16.start
  constraint midpoint L8 L20.start
  constraint coincident L4 L20.end
  constraint perpendicular L4 L20
  constraint midpoint L10 L21.start
  constraint midpoint L12 L21.end
  constraint perpendicular L12 L21
  constraint midpoint L14 L22.start
  constraint midpoint L16 L22.end
  constraint midpoint L18 L23.start
  constraint coincident L6 L23.end
  constraint perpendicular L6 L23
  constraint equal L20 L21
  constraint equal L21 L22
  constraint equal L22 L23
  constraint equal L9 L13
  constraint equal L13 L17
  constraint symmetric L8.start L24 L25.start
  constraint symmetric L8.end L24 L25.end
  constraint symmetric L9.end L24 L26.end
  constraint symmetric L10.end L24 L27.end
  constraint symmetric L12.start L24 L29.start
  constraint symmetric L12.end L24 L28.start
  constraint symmetric L13.end L24 L28.end
  constraint symmetric L14.end L24 L30.end
  constraint symmetric L16.start L24 L31.start
  constraint symmetric L16.end L24 L31.end
  constraint symmetric L17.end L24 L32.end
  constraint symmetric L18.end L24 L33.end
  constraint horizontal L34
  constraint vertical L35
  constraint vertical L36
  constraint coincident L4.end L5.start
  measures "d7" distance of L8.end L9.end
  measures "d8" distance of L8.start L8.end
  measures "d9" distance of L16.start L16.end
  measures "d13" distance of L34.start L2.end
extrude "Extruir2" add sketch "Boceto5" against normal blind 3 separate body contours L0 L1 L3 L6 L7 L18 | L1 L4 L5 L6 L9 L13 L17 L25 L26 L27 L28 L29 L30 L31 L32 L33 | L1 L3 L7 L14 L16 | L1 L3 L7 L10 L12 | L1 L2 L3 L4 L7 L8 | L2 L4 L34 L35 L36 | L37 L38 S0 L39 L40 S1 L41 L42 L43 L44 L45 L46 L47 L48 S2 L49 L50 S3 L51 L52 L53 L54 L55 L56 L57 L58 L59 L60 L61 L62 S4 L63 L64 L65 L66 S5 L67 L68 L69 L70 L71 L72 L73 L74 L75 L76 S6 L77 L78 L79 L80 | S7 L81 L82 L83 L84 L85 L86 L87 L88 L89 L90 L91 L92 S8 L93 L94 L95 L96 L97 L98 L99 L100 L101 L102 L103 L104 L105 L106 L107 L108 L109 L110 L111 L112 L113 L114 L115 L116 L117 L118 L119 L120 L121 L122 L123 L124 S9 S10 L125 L126 | L127 L128 L129 L130 L131 L132 L133 L134 L135 L136 L137 L138 L139 L140 L141 L142 L143 L144 L145 L146 S11 L147 L148 L149 L150 L151 L152 L153 L154 L155 L156 L157 L158 S12 L159 L160 L161 L162 L163 L164 L165 L166 L167 L168 L169 L170 L171 L172 L173 L174 S13 S14 L175 L176 L177 L178 | S15 L179 L180 S16 L181 L182 L183 L184 L185 L186 L187 L188 L189 L190 L191 L192 L193 L194 L195 L196 S17 L197 L198 L199 L200 L201 L202 L203 L204 S18 S19 L205 L206 L207 L208 S20 L209 L210 L211 L212 L213 L214 S21 L215 L216 L217 L218 S22 L219 L220 L221 L222 | S23 L223 L224 L225 L226 S24 L227 L228 L229 L230 L231 L232 L233 L234 L235 L236 L237 L238 L239 L240 L241 L242 L243 L244 S25 L245 L246 L247 L248 L249 L250 S26 L251 L252 L253 L254 L255 L256 L257 L258 L259 L260 S27 L261 L262 L263 L264 L265 L266 L267 L268 S28 | L269 L270 S29 L271 L272 L273 L274 L275 L276 L277 L278 L279 L280 S30 L281 L282 S31 L283 L284 S32 L285 L286 L287 L288 L289 L290 L291 L292 L293 L294 L295 L296 L297 L298 L299 L300 L301 L302 L303 L304 L305 L306 L307 L308 S33 L309 L310 L311 L312 | S34 L313 L314 S35 L315 L316 L317 L318 L319 L320 L321 L322 L323 L324 L325 L326 L327 L328 L329 L330 L331 L332 S36 L333 L334 L335 L336 L337 L338 L339 L340 S37 L341 L342 L343 L344 L345 L346 L347 L348 L349 L350 L351 L352 L353 L354 S38 L355 L356 S39 L357 L358 L359 L360 L361 L362 S40 | L363 L364 S41 L365 L366 S42 L367 L368 L369 L370 L371 L372 S43 L373 L374 L375 L376 S44 L377 L378 L379 L380 L381 L382 L383 L384 S45 L385 L386 L387 L388 L389 L390 L391 L392 S46 L393 L394 L395 L396 L397 L398 L399 L400 L401 L402 L403 L404 L405 L406 L407 L408 L409 L410 | S47 S48 L411 L412 L413 L414 S49 L415 L416 L417 L418 L419 L420 L421 L422 S50 L423 L424 S51 L425 L426 L427 L428 L429 L430 L431 L432 S52 S53 L433 L434 L435 L436 L437 L438 L439 L440 L441 L442 S54 L443 L444 L445 L446 S55 L447 L448 L449 L450 S56 | L451 L452 L453 L454 L455 L456 S57 L457 L458 L459 L460 L461 L462 L463 L464 L465 L466 S58 S59 S60 L467 L468 L469 L470 L471 L472 L473 L474 S61 L475 L476 L477 L478 L479 L480 L481 L482 L483 L484 L485 L486 L487 L488 S62 S63 S64 L489 L490 L491 L492 S65 | S66 L493 L494 L495 L496 L497 L498 L499 L500 L501 L502 L503 L504 L505 L506 L507 L508 L509 L510 L511 L512 L513 L514 L515 L516 L517 L518 L519 L520 L521 L522 L523 L524 L525 L526 S67 L527 L528 L529 L530 L531 L532 S68 L533 L534 S69 L535 L536 L537 L538 L539 L540 | L541 L542 S70 L543 L544 L545 L546 L547 L548 L549 L550 L551 L552 L553 L554 L555 L556 S71 L557 L558 L559 L560 L561 L562 L563 L564 L565 L566 L567 L568 L569 L570 S72 L571 L572 L573 L574 L575 L576 L577 L578 L579 L580 L581 L582 L583 L584 S73 L585 L586 L587 L588 | S74 S75 L589 L590 S76 L591 L592 L593 L594 L595 L596 S77 L597 L598 L599 L600 L601 L602 L603 L604 L605 L606 L607 L608 L609 L610 L611 L612 S78 L613 L614 L615 L616 L617 L618 L619 L620 S79 L621 L622 S80 L623 L624 L625 L626 | L627 L628 L629 L630 L631 L632 L633 L634 L635 L636 L637 L638 L639 L640 L641 L642 L643 L644 L645 L646 L647 L648 L649 L650 L651 L652 L653 L654 L655 L656 L657 L658 L659 L660 L661 L662 L663 L664 L665 L666 L667 L668 L669 L670 L671 L672 L673 L674 L675 L676 S81 L677 L678 L679 L680 L681 L682 | S82 L683 L684 S83 L685 L686 S84 L687 L688 L689 L690 L691 L692 L693 L694 L695 L696 L697 L698 S85 L699 L700 L701 L702 L703 L704 S86 L705 L706 L707 L708 L709 L710 L711 L712 L713 L714 L715 L716 S87 L717 L718 S88 L719 L720 L721 L722 | S89 L723 L724 L725 L726 L727 L728 S90 L729 L730 L731 L732 L733 L734 S91 S92 S93 L735 L736 L737 L738 L739 L740 L741 L742 L743 L744 L745 L746 L747 L748 L749 L750 L751 L752 L753 L754 L755 L756 L757 L758 S94 S95 L759 L760 L761 L762 L763 L764 L765 L766 | S96 L767 L768 L769 L770 L771 L772 L773 L774 S97 L775 L776 L777 L778 L779 L780 S98 L781 L782 S99 S100 L783 L784 L785 L786 L787 L788 L789 L790 L791 L792 L793 L794 L795 L796 L797 L798 L799 L800 L801 L802 L803 L804 L805 L806 L807 L808 S101 L809 L810 L811 L812 L813 L814 | S102 L815 L816 L817 L818 S103 L819 L820 L821 L822 L823 L824 L825 L826 L827 L828 L829 L830 L831 L832 L833 L834 L835 L836 S104 L837 L838 L839 L840 S105 L841 L842 S106 L843 L844 S107 L845 L846 L847 L848 L849 L850 S108 L851 L852 L853 L854 S109 L855 L856 | S110 L857 L858 L859 L860 S111 L861 L862 L863 L864 L865 L866 L867 L868 L869 L870 L871 L872 L873 L874 L875 L876 L877 L878 L879 L880 L881 L882 L883 L884 L885 L886 L887 L888 S112 L889 L890 S113 L891 L892 L893 L894 S114 L895 L896 L897 L898 S115 L899 L900 L901 L902 S116 | L903 L904 S117 L905 L906 S118 L907 L908 L909 L910 L911 L912 L913 L914 L915 L916 S119 L917 L918 L919 L920 L921 L922 L923 L924 L925 L926 L927 L928 L929 L930 L931 L932 L933 L934 S120 L935 L936 L937 L938 L939 L940 S121 L941 L942 L943 L944 | L945 L946 L947 L948 S122 L949 L950 L951 L952 L953 L954 S123 L955 L956 L957 L958 S124 S125 L959 L960 L961 L962 L963 L964 L965 L966 L967 L968 L969 L970 S126 L971 L972 L973 L974 S127 L975 L976 L977 L978 S128 L979 L980 L981 L982 L983 L984 | L985 L986 S129 S130 L987 L988 L989 L990 L991 L992 L993 L994 L995 L996 L997 L998 L999 L1000 L1001 L1002 S131 L1003 L1004 L1005 L1006 L1007 L1008 L1009 L1010 S132 L1011 L1012 L1013 L1014 L1015 L1016 L1017 L1018 L1019 L1020 L1021 L1022 S133 L1023 L1024 L1025 L1026 L1027 L1028 L1029 L1030 L1031 L1032 L1033 L1034 | L1035 L1036 L1037 L1038 S134 L1039 L1040 S135 L1041 L1042 L1043 L1044 L1045 L1046 L1047 L1048 L1049 L1050 L1051 L1052 L1053 L1054 S136 L1055 L1056 L1057 L1058 L1059 L1060 S137 L1061 L1062 L1063 L1064 L1065 L1066 S138 L1067 L1068 L1069 L1070 S139 L1071 L1072 S140 L1073 L1074 L1075 L1076 L1077 L1078 | S141 L1079 L1080 L1081 L1082 L1083 L1084 L1085 L1086 L1087 L1088 L1089 L1090 L1091 L1092 L1093 L1094 S142 L1095 L1096 L1097 L1098 S143 L1099 L1100 L1101 L1102 L1103 L1104 L1105 L1106 L1107 L1108 L1109 L1110 S144 L1111 L1112 L1113 L1114 S145 L1115 L1116 L1117 L1118 S146 L1119 L1120 L1121 L1122 L1123 L1124 L1125 L1126 makes body 2
combine "Combinar1" operation cut target body 1 tool bodies 2 keep tools
convert_to_sheet_metal "ConvertirAChapa1"
sketch "Boceto6" plane through (0, 0, 0) normal (0, 0, -1) x (1, 0, 0)
  line L0 (43, 37) -> (40, 37)
  line L1 (40, 37) -> (40, -15)
  line L2 (15, -40) -> (-15, -40)
  arc A0 (-40, -15) -> (-15, -40) centre (-15, -15) ccw
  line L3 (-40, -15) -> (-40, 37)
  line L4 (-40, 37) -> (-43, 37)
  line L5 (-43, 37) -> (-43, -15)
  arc A1 (-43, -15) -> (-15, -43) centre (-15, -15) ccw
  line L6 (-15, -43) -> (15, -43)
  line L7 (43, -15) -> (43, 37)
  line L8 (-43, 40) -> (43, 40)
  line L9 (43, 40) -> (43, -20)
  line L10 (20, -43) -> (-20, -43)
  line L11 (-43, -20) -> (-43, 40)
  arc A2 (-43, -20) -> (-20, -43) centre (-20, -20) ccw
  arc A3 (20, -43) -> (43, -20) centre (20, -20) ccw
  line L12 (40, 37) -> (40, -20)
  arc A4 (20, -40) -> (40, -20) centre (20, -20) ccw
  line L13 (20, -40) -> (-20, -40)
  arc A5 (-40, -20) -> (-20, -40) centre (-20, -20) ccw
  line L14 (-40, -20) -> (-40, 37)
  line L15 (-40, 37) -> (40, 37)
  line L16 (-31.7863, 40) -> (-16.7863, 40)
  line L17 (-16.7863, 40) -> (-16.7863, 37)
  line L18 (-16.7863, 37) -> (-31.7863, 37)
  line L19 (-31.7863, 37) -> (-31.7863, 40)
  line L20 (-5.5725, 40) -> (9.4275, 40)
  line L21 (9.4275, 40) -> (9.4275, 37)
  line L22 (9.4275, 37) -> (-5.5725, 37)
  line L23 (-5.5725, 37) -> (-5.5725, 40)
  line L24 (20.6412, 40) -> (35.6412, 40)
  line L25 (35.6412, 40) -> (35.6412, 37)
  line L26 (35.6412, 37) -> (20.6412, 37)
  line L27 (20.6412, 37) -> (20.6412, 40)
  line L28 (-31.7863, 38.5) -> (-43, 38.5) construction
  line L29 (-16.7863, 38.5) -> (-5.5725, 38.5) construction
  line L30 (9.4275, 38.5) -> (20.6412, 38.5) construction
  line L31 (35.6412, 38.5) -> (43, 46.9615) construction
  line L32 (-43, 30.0084) -> (-40, 30.0084)
  line L33 (-40, 30.0084) -> (-40, 15.0084)
  line L34 (-40, 15.0084) -> (-43, 15.0084)
  line L35 (-43, 15.0084) -> (-43, 30.0084)
  line L36 (-43, 5.0168) -> (-40, 5.0168)
  line L37 (-40, 5.0168) -> (-40, -9.9832)
  line L38 (-40, -9.9832) -> (-43, -9.9832)
  line L39 (-43, -9.9832) -> (-43, 5.0168)
  line L40 (-41.5, 30.0084) -> (-41.5, 40) construction
  line L41 (-41.5, 15.0084) -> (-41.5, 5.0168) construction
  line L42 (0, -2.5) -> (0, -20)
  line L43 (43, 30.0084) -> (40, 30.0084)
  line L44 (40, 30.0084) -> (40, 15.0084)
  line L45 (40, 15.0084) -> (43, 15.0084)
  line L46 (43, 5.0168) -> (40, 5.0168)
  line L47 (40, 5.0168) -> (40, -9.9832)
  line L48 (40, -9.9832) -> (43, -9.9832)
  line L49 (15, -40) -> (5, -40)
  line L50 (5, -40) -> (5, -43)
  line L51 (5, -43) -> (15, -43)
  line L52 (15, -43) -> (15, -40)
  line L53 (-15, -43) -> (-5, -43)
  line L54 (-5, -43) -> (-5, -40)
  line L55 (-5, -40) -> (-15, -40)
  line L56 (-15, -40) -> (-15, -43)
  arc A6 (15, -40) -> (40, -15) centre (15, -15) ccw
  arc A7 (15, -43) -> (43, -15) centre (15, -15) ccw
  point P0 (-43, 40)
  point P1 (43, 40)
  point P2 (41.5, 30.0084)
  dimension "d14" = 23
  dimension "d15" = 23
  dimension "d16" = 3
  dimension "d17" = 15
  dimension "d19" = 3
  dimension "d20" = 3
  dimension "d21" = 15
  constraint horizontal L8
  constraint vertical L9
  constraint horizontal L10
  constraint vertical L11
  constraint coincident P0 L8.start
  constraint coincident P1 L8.end
  constraint coincident A1.end L10
  constraint tangent L11 A2
  constraint tangent L10 A2
  constraint tangent L10 A3
  constraint tangent L9 A3
  constraint horizontal L16
  constraint vertical L17
  constraint horizontal L18
  constraint vertical L19
  constraint coincident L8 L16.start
  constraint horizontal L20
  constraint vertical L21
  constraint horizontal L22
  constraint vertical L23
  constraint coincident L8 L20.start
  constraint horizontal L24
  constraint vertical L25
  constraint horizontal L26
  constraint vertical L27
  constraint coincident L8 L24.start
  constraint midpoint L19 L28.start
  constraint coincident L11 L28.end
  constraint perpendicular L14 L28
  constraint midpoint L17 L29.start
  constraint midpoint L23 L29.end
  constraint midpoint L21 L30.start
  constraint midpoint L27 L30.end
  constraint perpendicular L27 L30
  constraint midpoint L25 L31.start
  constraint coincident L9 L31.end
  constraint equal L30 L31
  constraint equal L29 L30
  constraint equal L28 L29
  constraint equal L18 L22
  constraint equal L22 L26
  constraint horizontal L32
  constraint vertical L33
  constraint horizontal L34
  constraint vertical L35
  constraint coincident L14 L33.end
  constraint coincident L5 L32.start
  constraint horizontal L36
  constraint vertical L37
  constraint horizontal L38
  constraint vertical L39
  constraint coincident L14 L37.end
  constraint coincident L11 L36.start
  constraint midpoint L32 L40.start
  constraint coincident L8 L40.end
  constraint perpendicular L8 L40
  constraint midpoint L34 L41.start
  constraint midpoint L36 L41.end
  constraint equal L40 L41
  constraint equal L33 L37
  constraint symmetric L32.start L42 L43.start
  constraint symmetric L32.end L42 L43.end
  constraint symmetric L33.end L42 L44.end
  constraint symmetric L34.end L42 L45.end
  constraint symmetric L36.start L42 L46.start
  constraint symmetric L36.end L42 L46.end
  constraint symmetric L37.end L42 L47.end
  constraint symmetric L38.end L42 L48.end
  constraint symmetric L40.start L42 P2
  constraint horizontal L49
  constraint vertical L50
  constraint horizontal L51
  constraint vertical L52
  constraint coincident L6 L50.end
  constraint coincident L2.start L49.start
  constraint horizontal L53
  constraint vertical L54
  constraint horizontal L55
  constraint vertical L56
  constraint coincident L13 L54.end
  constraint coincident A1.end L6.start
  measures "d14" radius of A2
  measures "d15" radius of A3
  measures "d17" distance of L17.end L18.end
  measures "d19" distance of L24.end L25.end
  measures "d20" distance of L16.start L18.end
extrude "Extruir3" add sketch "Boceto6" against normal blind 3 separate body contours L0 L1 L7 L9 L12 L43 | L0 L8 L9 L15 L25 | L1 L2 A0 L3 L12 L13 L14 L15 L18 L22 L26 L33 L37 L44 L47 L49 L55 A6 | L1 L7 L9 L12 L45 L46 | L8 L15 L21 L27 | L1 L7 L9 L12 A4 L13 L48 L52 A7 | L8 L15 L17 L23 | L12 A4 L13 A6 | L4 L8 L11 L15 L19 | L2 L6 L10 L13 L50 L54 | L3 L4 L5 L11 L14 L32 | L3 L5 A1 L11 L13 A5 L14 L38 L56 | A0 L13 A5 L14 | L3 L5 L11 L14 L34 L36 makes body 3
combine "Combinar2" operation cut target body 1 tool bodies 3 keep tools
combine "Combinar3" operation cut target body 2 tool bodies 3 keep tools